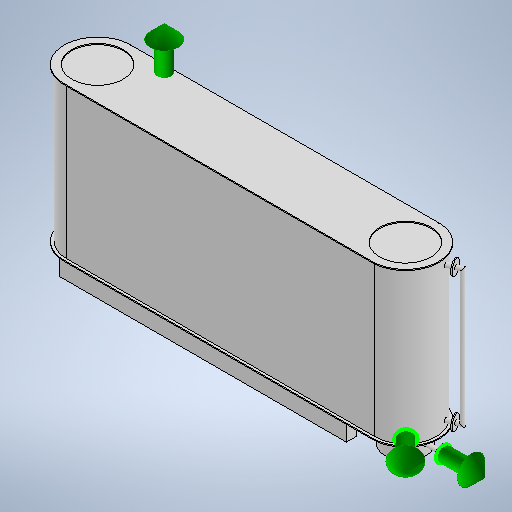
# Autodesk Inventor part: GNG НаOCl tank
Saved by Autodesk Inventor 2025 (Build 290162010, 162A)
## iProperties
Created: 2025-09-24
Part Number: GNG НаOCl tank
Material: Generic
Document SubType Name: Modeling
Designer: admin
Density: 1 g/cm^3
Appearance: Default
Mass: 3.26431e+06 g
Surface Area: 197551 cm^2
Volume: 3.26431e+06 cm^3
Author: admin
Autodesk Inventor part; units mm, degrees
sketch "Sketch1" plane through (0, 0, 0) normal (0, 0, 1) x (1, 0, 0)
  line L0 (-1500, 0) -> (1500, 0) construction
  line L1 (-1500, -300) -> (1500, -300)
  line L2 (1500, 300) -> (-1500, 300)
  arc A0 (-1500, 300) -> (-1500, -300) centre (-1500, 0) ccw
  arc A1 (1500, -300) -> (1500, 300) centre (1500, 0) ccw
  point P0 (0, 0)
  point P1 (0, 0)
  dimension "d0" = 3000
  dimension "d1" = 600
  constraints: 8 end point, 4 point on circle, 4 tangent, 2 centre point, 1 coincident, 1 horizontal, 1 midpoint, 1 parallel
  measures "d0" distance of L0.start L0.end
  measures "d1" diameter of A1
extrude "Extrusion1" add sketch "Sketch1" along normal blind 1500
sketch "Sketch2" plane through (0, 0, 1500) normal (0, 0, 1) x (1, 0, 0)
  arc A0 (1500, -300) -> (1500, 300) centre (1500, 0) ccw projected
  line L0 (1500, 300) -> (-1500, 300) projected
  arc A1 (-1500, 300) -> (-1500, -300) centre (-1500, 0) ccw projected
  line L1 (-1500, -300) -> (1500, -300) projected
  line L2 (-1500, 325) -> (1500, 325)
  arc A2 (1500, -325) -> (1500, 325) centre (1500, 0) ccw
  line L3 (1500, -325) -> (-1500, -325)
  arc A3 (-1500, 325) -> (-1500, -325) centre (-1500, 0) ccw
  point P0 (0, 0)
  dimension "d4" = 25
  constraints: 4 end point, 4 point on circle, 2 centre point, 3 other
  measures "d4" distance between parallel lines of L0 L2
extrude "Extrusion2" add sketch "Sketch2" against normal blind 10
sketch "Sketch3" plane through (0, 0, 0) normal (0, 0, -1) x (-1, 0, 0)
  arc A0 (-1500, 300) -> (-1500, -300) centre (-1500, 0) ccw projected
  line L0 (1500, -300) -> (-1500, -300) projected
  arc A1 (1500, -300) -> (1500, 300) centre (1500, 0) ccw projected
  line L1 (-1500, 300) -> (1500, 300) projected
  arc A2 (-1500, 325) -> (-1500, -325) centre (-1500, 0) ccw
  line L2 (-1500, 325) -> (1500, 325)
  arc A3 (1500, -325) -> (1500, 325) centre (1500, 0) ccw
  line L3 (1500, -325) -> (-1500, -325)
  point P0 (0, 0)
  dimension "d7" = 25
  constraints: 4 end point, 4 point on circle, 2 centre point, 3 other
  measures "d7" distance between parallel lines of L0 L3
extrude "Extrusion3" add sketch "Sketch3" against normal blind 10
sketch "Sketch4" plane through (0, 0, 0) normal (0, 0, -1) x (-1, 0, 0)
  circle A0 centre (-1500, 0) radius 200
  arc A1 (-1500, 300) -> (-1500, -300) centre (-1500, 0) ccw projected
  arc A2 (-1500, 300) -> (-1500, -300) centre (-1500, 0) ccw projected
  point P0 (0, 0)
  dimension "d10" = 400
  dimension "d71" = 0
  constraints: 1 centre point
  measures "d10" diameter of A0
  measures "d71" distance of A0.centre A1.centre
extrude "Extrusion4" add sketch "Sketch4" along normal blind 200
ref_plane "Work Plane1" through (1500, -300, 0) normal (-1, 0, 0) x (0, 0, 1)
sketch "Sketch5" plane through (1500, -300, 0) normal (-1, 0, 0) x (0, 0, 1)
  line L0 (-200, 500) -> (-200, 100) projected
  line L1 (0, 100) -> (0, 500) projected
  circle A0 centre (-100, 300) radius 20
  point P0 (0, 300)
  point P1 (0, 300)
  dimension "d13" = 40
  dimension "d14" = 100
  constraints: 1 centre point, 1 horizontal alignment, 1 midpoint
  measures "d13" diameter of A0
  measures "d14" distance from line of A0.centre L0
extrude "Extrusion5" add sketch "Sketch5" against normal blind 365
sketch "Sketch6" plane through (1865, 0, -100) normal (1, 0, 0) x (0, 0, -1)
  circle A0 centre (0, 0) radius 20
  circle A1 centre (0, 0) radius 72.5
  line L0 (-100, -325) -> (-100, 325)
  line L1 (72.5, 0) -> (72.5, -294.97794)
  point P0 (-100, 0)
  dimension "d18" = 145
  dimension "d40" = 172.5
  constraints: 2 end point, 2 vertical, 1 coincident, 1 horizontal alignment, 2 other
  measures "d40" distance between parallel lines of L1 L0
extrude "Extrusion6" add sketch "Sketch6" against normal blind 10
sketch "Sketch7" plane through (0, 0, 1500) normal (0, 0, 1) x (1, 0, 0)
  line L0 (1500, 325) -> (-1500, 325)
  arc A0 (-1500, 325) -> (-1500, -325) centre (-1500, 0) ccw
  line L1 (-1500, -325) -> (1500, -325)
  arc A1 (1500, -325) -> (1500, 325) centre (1500, 0) ccw
  line L2 (1500, 0) -> (1825, 0)
  line L3 (1500, 0) -> (1800.260848, 124.372116)
  line L4 (1500, 0) -> (1729.809704, -229.809704)
  point P0 (0, 0)
  dimension "d21" = 22.5
  dimension "d23" = 45
  constraints: 6 end point, 3 point on circle
  measures "d21" angle of L2 L3
  measures "d23" angle of L2 L4
ref_plane "Work Plane2" through (1800.260848, 124.372116, 1500) normal (0.9238795, 0.3826834, 0) x (-0.3826834, 0.9238795, 0)
ref_plane "Work Plane3" through (1729.809704, -229.809704, 1500) normal (0.7071068, -0.7071068, 0) x (0.7071068, 0.7071068, 0)
sketch "Sketch8" plane through (1800.260848, 124.372116, 1500) normal (0.9238795, 0.3826834, 0) x (-0.3826834, 0.9238795, 0)
  line L0 (277.16386, -1490) -> (277.16386, -10)
  line L1 (-277.16386, -1490) -> (-277.16386, -10)
  circle A0 centre (0, -110) radius 20
  circle A1 centre (0, -1420) radius 20
  line L2 (-277.16386, -1490) -> (277.16386, -1490)
  line L3 (277.16386, -10) -> (-277.16386, -10)
  point P0 (574.025149, -1500)
  point P1 (0, 0)
  point P2 (0, 0)
  point P3 (0, 0)
  dimension "d24" = 40
  constraints: 2 centre point, 2 vertical alignment, 1 equal radius
  measures "d24" diameter of A0
extrude "Extrusion7" add sketch "Sketch8" along normal blind 50 and the other way blind 100 contours A0 | A1
sketch "Sketch9" plane through (1729.809704, -229.809704, 1500) normal (0.7071068, -0.7071068, 0) x (0.7071068, 0.7071068, 0)
  line L0 (212.132034, -1490) -> (212.132034, -10)
  line L1 (-212.132034, -1490) -> (-212.132034, -10)
  circle A0 centre (0, -1390) radius 31.5
  line L2 (-212.132034, -1490) -> (212.132034, -1490)
  line L3 (212.132034, -10) -> (-212.132034, -10)
  point P0 (-1060.660172, -1500)
  point P1 (0, 0)
  point P2 (0, 0)
  point P3 (0, 0)
  dimension "d31" = 63
  constraints: 1 centre point, 1 vertical alignment
  measures "d31" diameter of A0
extrude "Extrusion8" add sketch "Sketch9" along normal blind 50 and the other way blind 100 contours A0
sketch "Sketch10" plane through (1765.165043, -265.165043, 110) normal (0.7071068, -0.7071068, 0) x (-0.7071068, -0.7071068, 0)
  circle A0 centre (0, 0) radius 31.5 projected
  circle A1 centre (0, 0) radius 80
  point P0 (1060.660172, 110)
  dimension "d37" = 160
  constraints: 1 centre point, 1 coincident
  measures "d37" diameter of A1
extrude "Extrusion9" add sketch "Sketch10" against normal blind 10
sketch "Sketch13" plane through (1846.454825, 143.506287, 80) normal (0.9238795, 0.3826834, 0) x (0, 0, -1)
  circle A0 centre (0, 0) radius 20 projected
  circle A1 centre (-1310, 0) radius 20 projected
  circle A2 centre (-1310, 0) radius 67.5
  circle A3 centre (0, 0) radius 67.5
  point P0 (80, 574.025149)
  dimension "d44" = 135
  dimension "d45" = 135
  constraints: 2 centre point, 2 coincident
  measures "d44" diameter of A2
  measures "d45" diameter of A3
extrude "Extrusion10" add sketch "Sketch13" against normal blind 10
sketch "Sketch14" plane through (0, 0, 1500) normal (0, 0, 1) x (1, 0, 0)
  arc A0 (-1500, 300) -> (-1500, -300) centre (-1500, 0) ccw projected
  circle A1 centre (-1500, 0) radius 250
  arc A2 (1500, -300) -> (1500, 300) centre (1500, 0) ccw projected
  circle A3 centre (1500, 0) radius 250
  point P0 (0, 0)
  dimension "d48" = 500
  dimension "d49" = 500
  constraints: 2 centre point, 2 coincident
  measures "d48" diameter of A1
  measures "d49" diameter of A3
extrude "Extrusion11" cut sketch "Sketch14" against normal blind 10
sketch "Sketch15" plane through (0, 0, 0) normal (0, 0, -1) x (-1, 0, 0)
  line L0 (-1200, -175) -> (1600, -175)
  line L1 (1600, -175) -> (1600, -275)
  line L2 (1600, -275) -> (-1200, -275)
  line L3 (-1200, -275) -> (-1200, -175)
  line L4 (-1200, 175) -> (1600, 175)
  line L5 (1600, 175) -> (1600, 275)
  line L6 (1600, 275) -> (-1200, 275)
  line L7 (-1200, 275) -> (-1200, 175)
  line L8 (0, 0) -> (1601.478947, 0)
  line L9 (-1500, -325) -> (1500, -325)
  line L10 (1500, 325) -> (-1500, 325)
  point P0 (200, -275)
  point P1 (0, -325)
  point P2 (0, 325)
  dimension "d52" = 100
  dimension "d53" = 550
  dimension "d59" = 1200
  dimension "d60" = 1600
  constraints: 18 end point, 4 parallel, 3 horizontal, 3 midpoint, 2 equal length, 2 perpendicular, 1 collinear, 1 other
  measures "d52" distance of L0.end L1.end
  measures "d53" distance between parallel lines of L6 L2
  measures "d59" distance from line of L3 point (0, -325)
  measures "d60" horizontal distance of point (0, 325) L5.end
extrude "Extrusion12" add sketch "Sketch15" along normal blind 200
sketch "Sketch16" plane through (0, 0, 1500) normal (0, 0, 1) x (1, 0, 0)
  circle A0 centre (-1100, -250) radius 25
  circle A1 centre (-1100, 250) radius 25
  line L0 (0, 0) -> (-789.655633, 0)
  dimension "d62" = 50
  dimension "d63" = 1100
  dimension "d64" = 250
  constraints: 2 centre point, 2 end point, 1 horizontal, 1 other
  measures "d62" diameter of A0
  measures "d63" horizontal distance of L0.start A0.centre
  measures "d64" vertical distance of A0.centre L0.start
extrude "Extrusion13" add sketch "Sketch16" along normal blind 10 contours A1
sketch "Sketch19" plane through (1846.454825, 143.506287, 1390) normal (0.9238795, 0.3826834, 0) x (0, 0, -1)
  circle A0 centre (0, 0) radius 67.5 construction
  circle A1 centre (0, 0) radius 20 projected
  line L0 (0, 0) -> (67.5, 0) construction
  point P0 (1390, 574.025149)
  constraints: 2 end point, 1 horizontal, 1 horizontal alignment, 1 other
ref_plane "Work Plane7" through (1500, 0, 1500) normal (-0.3826834, 0.9238795, 0) x (0.9238795, 0.3826834, 0)
sketch "Sketch20" plane through (1500, 0, 1500) normal (-0.3826834, 0.9238795, 0) x (0.9238795, 0.3826834, 0)
  line L0 (375, 1352.5) -> (375, 1487.5) construction
  line L1 (375, 42.5) -> (375, 177.5) construction
  line L2 (375, 110) -> (425, 110)
  line L3 (425, 110) -> (425, 1420)
  line L4 (425, 1420) -> (375, 1420)
  point P0 (-1385.819299, 1500)
  dimension "d68" = 50
  constraints: 6 end point, 2 midpoint, 1 horizontal, 1 parallel, 1 perpendicular
  measures "d68" distance of L2.start L2.end
sweep "Sweep1" add profiles "Sketch19" path "Sketch20"
equation "\"d49\" = d48"
body "Solid1"
